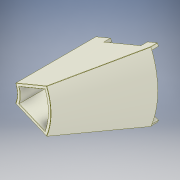
# Autodesk Inventor part: rear curved panel
Saved by Autodesk Inventor 2019 (Build 230136000, 136)
## iProperties
Created: 2019-01-04
Part Number: rear curved panel
Material: Phenolic Resin
Document SubType Name: Sheet Metal
Designer: gaincarlo
Density: 1.38 g/cm^3
Appearance: Smooth - Ivory
Sheet Metal Rule: Default_mm
Author: gaincarlo
Autodesk Inventor part; units mm, degrees
ref_plane "Work Plane1" through (0, 0, 600) normal (0, 0, 1) x (1, 0, 0)
sketch "Sketch1" plane through (0, 0, 600) normal (0, 0, 1) x (1, 0, 0)
  line L0 (-203.901986, -66.969601) -> (27.067897, -162.640459)
  arc A0 (-203.901986, -66.969601) -> (-203.901986, 66.969601) centre (-365.580904, 0) ccw
  line L1 (-203.901986, 66.969601) -> (27.067897, 162.640459)
  line L2 (-365.580904, 0) -> (376.715348, 0) construction
  arc A1 (27.067897, -162.640459) -> (27.067897, 162.640459) centre (-365.580904, 0) ccw
  point P0 (0, 0)
  dimension "d1" = 22.5
  dimension "d2" = 22.5
  dimension "d3" = 250
  dimension "d6" = 350
  constraints: 6 end point, 4 point on circle, 2 centre point, 1 coincident, 1 horizontal
  measures "d1" angle of L2 L0
  measures "d2" angle of L1 L2
  measures "d3" radial gap between concentric circles of A1 A0
  measures "d6" diameter of A0
ref_plane "Work Plane2" through (0, 0, 50) normal (0, 0, 1) x (1, 0, 0)
sketch "Sketch2" plane through (0, 0, 50) normal (0, 0, 1) x (1, 0, 0)
  circle A0 centre (-365.580904, 0) radius 175 construction
  arc A1 (258.03778, -258.311317) -> (258.03778, 258.311317) centre (-365.580904, 0) ccw
  line L0 (-203.901986, -66.969601) -> (258.03778, -258.311317)
  line L1 (-203.901986, 66.969601) -> (258.03778, 258.311317)
  arc A2 (-203.901986, -66.969601) -> (-203.901986, 66.969601) centre (-365.580904, 0) ccw
  dimension "d5" = 500
  constraints: 6 point on circle, 4 end point, 2 centre point, 1 coincident
  measures "d5" radial gap between concentric circles of A1 A0
loft "Loft1" add profiles "Sketch2", "Sketch1"
sketch "Sketch3" plane through (-365.580904, 0, 600) normal (0, 0, 1) x (1, 0, 0)
  line L0 (392.648801, -162.640459) -> (161.678918, -66.969601)
  arc A0 (161.678918, -66.969601) -> (161.678918, 66.969601) centre (0, 0) ccw
  line L1 (161.678918, 66.969601) -> (392.648801, 162.640459)
  arc A1 (392.648801, -162.640459) -> (392.648801, 162.640459) centre (0, 0) ccw
  line L2 (186.860104, -55.752145) -> (381.368364, -136.320105)
  arc A2 (381.368364, -136.320105) -> (381.368364, 136.320105) centre (0, 0) ccw
  line L3 (381.368364, 136.320105) -> (186.860104, 55.752145)
  arc A3 (186.860104, -55.752145) -> (186.860104, 55.752145) centre (0, 0) ccw
  point P0 (365.580904, 0)
  dimension "d11" = 20
  constraints: 4 end point, 4 point on circle, 2 centre point, 3 other
  measures "d11" distance between parallel lines of L0 L2
extrude "Extrusion1" cut sketch "Sketch3" against normal blind 250 contours A3 L3 A2 L2
sketch "Sketch4" plane through (-365.580904, 0, 50) normal (0, 0, -1) x (-1, 0, 0)
  line L0 (-161.678918, -66.969601) -> (-623.618684, -258.311317) construction
  arc A0 (-623.618684, 258.311317) -> (-623.618684, -258.311317) centre (0, 0) ccw construction
  line L1 (-623.618684, 258.311317) -> (-161.678918, 66.969601) construction
  arc A1 (-161.678918, 66.969601) -> (-161.678918, -66.969601) centre (0, 0) ccw construction
  line L2 (-186.860104, 55.752145) -> (-381.368364, 136.320105) construction
  arc A2 (-186.860104, 55.752145) -> (-186.860104, -55.752145) centre (0, 0) ccw construction
  line L3 (-381.368364, -136.320105) -> (-186.860104, -55.752145) construction
  line L4 (-272.544462, 112.891613) -> (-280.198131, 94.414022)
  line L5 (-173.853387, 20) -> (-193.971647, 20)
  line L6 (-272.544462, 112.891613) -> (-161.678918, 66.969601)
  line L7 (-186.860104, 55.752145) -> (-381.368364, 136.320105) construction
  line L8 (-280.198131, 94.414022) -> (-186.860104, 55.752145)
  arc A3 (-161.678918, 66.969601) -> (-161.678918, -66.969601) centre (0, 0) ccw construction
  arc A4 (-161.678918, 66.969601) -> (-173.853387, 20) centre (0, 0) ccw
  arc A5 (-186.860104, 55.752145) -> (-186.860104, -55.752145) centre (0, 0) ccw construction
  arc A6 (-186.860104, 55.752145) -> (-193.971647, 20) centre (0, 0) ccw
  line L9 (-549.708322, 227.696642) -> (-557.36199, 209.219052)
  line L10 (-557.36199, 209.219052) -> (-630.998551, 239.720314)
  line L11 (-161.678918, 66.969601) -> (-623.618684, 258.311317) construction
  arc A7 (-623.618684, 258.311317) -> (-623.618684, -258.311317) centre (0, 0) ccw construction
  arc A8 (-623.618684, 258.311317) -> (-630.998551, 239.720314) centre (0, 0) ccw
  line L12 (-623.618684, 258.311317) -> (-392.648801, 162.640459) construction
  line L13 (-623.618684, 258.311317) -> (-549.708322, 227.696642)
  point P0 (-365.580904, 0)
  dimension "d14" = 120
  dimension "d15" = 20
  dimension "d18" = 80
  dimension "d20" = 20
  constraints: 14 end point, 10 point on circle, 4 perpendicular, 3 centre point, 3 coincident, 3 point on line, 1 collinear, 1 horizontal
  measures "d14" distance from line of L4 L1.end
  measures "d15" distance from line of A0.centre L5
  measures "d18" distance from line of L9 L1.start
  measures "d20" distance of L9.start L9.end
extrude "Extrusion2" add sketch "Sketch4" along normal blind 50
mirror "Mirror1" about plane through (0, 0, 0) normal (0, 1, 0) of "Extrusion2"
ref_plane "Work Plane3" through (0, 0, 300) normal (0, 0, 1) x (1, 0, 0)
sketch "Sketch5" plane through (0, 0, 300) normal (0, 0, 1) x (1, 0, 0)
  line L0 (153.05147, -214.824563) -> (-203.901986, -66.969601) construction
  arc A0 (-203.901986, -66.969601) -> (-203.901986, 66.969601) centre (-365.580904, 0) ccw construction
  line L1 (-203.901986, 66.969601) -> (153.05147, 214.824563) construction
  arc A1 (153.05147, -214.824563) -> (153.05147, 214.824563) centre (-365.580904, 0) ccw construction
  line L2 (-166.744101, -49.889135) -> (136.032549, -175.303329)
  arc A2 (136.032549, -175.303329) -> (136.032549, 175.303329) centre (-365.580904, 0) ccw construction
  line L3 (136.032549, 175.303329) -> (-166.744101, 49.889135)
  arc A3 (-166.744101, -49.889135) -> (-166.744101, 49.889135) centre (-365.580904, 0) ccw construction
  line L4 (136.032549, -175.303329) -> (136.032549, 175.303329)
  line L5 (-166.744101, -49.889135) -> (-166.744101, 49.889135)
  point P0 (0, 0)
  dimension "d22" = 30
  constraints: 8 end point, 4 point on circle, 2 centre point, 2 vertical, 3 other
  measures "d22" distance between parallel lines of L0 L2
sketch "Sketch6" plane through (-171.609257, 20, 50) normal (0, 0, -1) x (-1, 0, 0)
  line L0 (-78.572815, -132.891613) -> (-86.226483, -114.414022) construction
  line L1 (-86.226483, -114.414022) -> (7.111544, -75.752145) construction
  arc A0 (0, -40) -> (7.111544, -75.752145) centre (193.971647, -20) ccw construction
  line L2 (0, -40) -> (20.118261, -40) construction
  arc A1 (20.118261, 0) -> (20.118261, -40) centre (193.971647, -20) ccw construction
  line L3 (20.118261, 0) -> (0, 0) construction
  arc A2 (7.111544, 35.752145) -> (0, 0) centre (193.971647, -20) ccw construction
  line L4 (7.111544, 35.752145) -> (-86.226483, 74.414022) construction
  line L5 (-86.226483, 74.414022) -> (-78.572815, 92.891613) construction
  line L6 (-78.572815, 92.891613) -> (-355.736674, 207.696642) construction
  line L7 (-355.736674, 207.696642) -> (-363.390343, 189.219052) construction
  line L8 (-363.390343, 189.219052) -> (-437.026903, 219.720314) construction
  arc A3 (-437.026903, 219.720314) -> (-437.026903, -259.720314) centre (193.971647, -20) ccw construction
  line L9 (-437.026903, -259.720314) -> (-363.390343, -229.219052) construction
  line L10 (-363.390343, -229.219052) -> (-355.736674, -247.696642) construction
  line L11 (-355.736674, -247.696642) -> (-78.572815, -132.891613) construction
  line L12 (-355.736674, 207.696642) -> (-363.390343, 189.219052) construction
  line L13 (-363.390343, 189.219052) -> (-437.026903, 219.720314) construction
  arc A4 (-429.647037, 238.311317) -> (-437.026903, 219.720314) centre (193.971647, -20) ccw construction
  line L14 (-429.647037, 238.311317) -> (-355.736674, 207.696642) construction
  line L15 (-355.736674, 207.696642) -> (-78.572815, 92.891613) construction
  line L16 (-78.572815, 92.891613) -> (32.292729, 46.969601) construction
  arc A5 (32.292729, 46.969601) -> (20.118261, 0) centre (193.971647, -20) ccw construction
  arc A6 (20.118261, 0) -> (20.118261, -40) centre (193.971647, -20) ccw construction
  arc A7 (20.118261, -40) -> (32.292729, -86.969601) centre (193.971647, -20) ccw construction
  line L17 (32.292729, -86.969601) -> (-78.572815, -132.891613) construction
  line L18 (-78.572815, -132.891613) -> (-86.226483, -114.414022) construction
  line L19 (-86.226483, -114.414022) -> (7.111544, -75.752145) construction
  arc A8 (0, -40) -> (7.111544, -75.752145) centre (193.971647, -20) ccw construction
  line L20 (0, -40) -> (20.118261, -40) construction
  arc A9 (-437.026903, 219.720314) -> (-437.026903, -259.720314) centre (193.971647, -20) ccw construction
  arc A10 (-437.026903, -259.720314) -> (-429.647037, -278.311317) centre (193.971647, -20) ccw construction
  line L21 (-355.736674, -247.696642) -> (-429.647037, -278.311317) construction
  line L22 (-363.390343, -229.219052) -> (-355.736674, -247.696642) construction
  line L23 (-437.026903, -259.720314) -> (-363.390343, -229.219052) construction
  line L24 (-86.226483, 74.414022) -> (-78.572815, 92.891613) construction
  line L25 (7.111544, 35.752145) -> (-86.226483, 74.414022) construction
  arc A11 (7.111544, 35.752145) -> (0, 0) centre (193.971647, -20) ccw construction
  line L26 (20.118261, 0) -> (0, 0) construction
  line L27 (-78.572815, -132.891613) -> (-355.736674, -247.696642) construction
  line L28 (-412.766238, -238.847295) -> (-4.865156, -69.889135)
  line L29 (-4.865156, 29.889135) -> (-412.766238, 198.847295)
  line L30 (-355.736674, 207.696642) -> (-363.390343, 189.219052) construction
  line L31 (-363.390343, 189.219052) -> (-437.026903, 219.720314) construction
  arc A12 (-429.647037, 238.311317) -> (-437.026903, 219.720314) centre (193.971647, -20) ccw construction
  line L32 (-429.647037, 238.311317) -> (-355.736674, 207.696642) construction
  line L33 (-355.736674, 207.696642) -> (-78.572815, 92.891613) construction
  line L34 (-78.572815, 92.891613) -> (32.292729, 46.969601) construction
  arc A13 (32.292729, 46.969601) -> (20.118261, 0) centre (193.971647, -20) ccw construction
  arc A14 (20.118261, 0) -> (20.118261, -40) centre (193.971647, -20) ccw construction
  arc A15 (20.118261, -40) -> (32.292729, -86.969601) centre (193.971647, -20) ccw construction
  line L35 (32.292729, -86.969601) -> (-78.572815, -132.891613) construction
  line L36 (-78.572815, -132.891613) -> (-86.226483, -114.414022) construction
  line L37 (-86.226483, -114.414022) -> (7.111544, -75.752145) construction
  arc A16 (0, -40) -> (7.111544, -75.752145) centre (193.971647, -20) ccw construction
  line L38 (0, -40) -> (20.118261, -40) construction
  arc A17 (-437.026903, 219.720314) -> (-437.026903, -259.720314) centre (193.971647, -20) ccw construction
  arc A18 (-437.026903, -259.720314) -> (-429.647037, -278.311317) centre (193.971647, -20) ccw construction
  line L39 (-355.736674, -247.696642) -> (-429.647037, -278.311317) construction
  line L40 (-363.390343, -229.219052) -> (-355.736674, -247.696642) construction
  line L41 (-437.026903, -259.720314) -> (-363.390343, -229.219052) construction
  line L42 (-86.226483, 74.414022) -> (-78.572815, 92.891613) construction
  line L43 (7.111544, 35.752145) -> (-86.226483, 74.414022) construction
  arc A19 (7.111544, 35.752145) -> (0, 0) centre (193.971647, -20) ccw construction
  line L44 (20.118261, 0) -> (0, 0) construction
  line L45 (-78.572815, -132.891613) -> (-355.736674, -247.696642) construction
  line L46 (-355.736674, 207.696642) -> (-363.390343, 189.219052) construction
  line L47 (-363.390343, 189.219052) -> (-437.026903, 219.720314) construction
  arc A20 (-429.647037, 238.311317) -> (-437.026903, 219.720314) centre (193.971647, -20) ccw construction
  line L48 (-429.647037, 238.311317) -> (-355.736674, 207.696642) construction
  line L49 (-355.736674, 207.696642) -> (-78.572815, 92.891613) construction
  line L50 (-78.572815, 92.891613) -> (32.292729, 46.969601) construction
  arc A21 (32.292729, 46.969601) -> (20.118261, 0) centre (193.971647, -20) ccw construction
  arc A22 (20.118261, 0) -> (20.118261, -40) centre (193.971647, -20) ccw construction
  arc A23 (20.118261, -40) -> (32.292729, -86.969601) centre (193.971647, -20) ccw construction
  line L51 (32.292729, -86.969601) -> (-78.572815, -132.891613) construction
  line L52 (-78.572815, -132.891613) -> (-86.226483, -114.414022) construction
  line L53 (-86.226483, -114.414022) -> (7.111544, -75.752145) construction
  arc A24 (0, -40) -> (7.111544, -75.752145) centre (193.971647, -20) ccw construction
  line L54 (0, -40) -> (20.118261, -40) construction
  arc A25 (-437.026903, 219.720314) -> (-437.026903, -259.720314) centre (193.971647, -20) ccw construction
  arc A26 (-437.026903, -259.720314) -> (-429.647037, -278.311317) centre (193.971647, -20) ccw construction
  line L55 (-355.736674, -247.696642) -> (-429.647037, -278.311317) construction
  line L56 (-363.390343, -229.219052) -> (-355.736674, -247.696642) construction
  line L57 (-437.026903, -259.720314) -> (-363.390343, -229.219052) construction
  line L58 (-86.226483, 74.414022) -> (-78.572815, 92.891613) construction
  line L59 (7.111544, 35.752145) -> (-86.226483, 74.414022) construction
  arc A27 (7.111544, 35.752145) -> (0, 0) centre (193.971647, -20) ccw construction
  line L60 (20.118261, 0) -> (0, 0) construction
  line L61 (-78.572815, -132.891613) -> (-355.736674, -247.696642) construction
  arc A28 (-9.685177, -43.428571) -> (-4.865156, -69.889135) centre (193.971647, -20) ccw construction
  arc A29 (-9.685177, 3.428571) -> (-9.685177, -43.428571) centre (193.971647, -20) ccw construction
  arc A30 (-409.297777, -248.234533) -> (-408.982523, -249.066077) centre (193.971647, -20) ccw construction
  arc A31 (-408.982523, 209.066077) -> (-409.297777, 208.234533) centre (193.971647, -20) ccw construction
  arc A32 (-412.766238, 198.847295) -> (-412.766238, -238.847295) centre (193.971647, -20) ccw construction
  arc A33 (-4.865156, 29.889135) -> (-9.685177, 3.428571) centre (193.971647, -20) ccw construction
  line L62 (-4.865156, -69.889135) -> (-4.865156, 29.889135)
  line L63 (-412.766238, -238.847295) -> (-412.766238, 198.847295)
  point P0 (-171.609257, -20)
  dimension "d24" = 30
  dimension "d25" = 30
  dimension "d26" = 30
  dimension "d27" = 30
  constraints: 12 point on circle, 8 end point, 6 centre point, 2 parallel, 2 point on line, 1 vertical
  measures "d24" distance between parallel lines of L28 L27
  measures "d25" distance between parallel lines of L29 L6
  measures "d26" radial gap between concentric circles of A29 A1
  measures "d27" radial gap between concentric circles of A28 A7
loft "Loft2" cut profiles "Sketch5", "Sketch6"
fillet "Fillet1" radius 2 16 edges at (-203.902, -66.9696, 325) (-203.902, -66.9696, 25) (-203.902, 66.9696, 325) (-203.902, 66.9696, 25) (142.5528, -210.4759, 325) (142.5528, 210.4759, 325) (-88.417, 114.805, 600) (-190.5809, 0, 600) (-88.417, -114.805, 600) (59.4191, 0, 600) (39.4191, 0, 600) (-81.4667, 96.0361, 600) (-170.5809, 0, 600) (-81.4667, -96.0361, 600) (258.0378, 258.3113, 25) (258.0378, -258.3113, 25)
thicken "Thicken1" operation new thickness 2 both sides no extend neighbours no toward (0.8502244, -0.3254007, 0.4138029) faces at (148.215845, -196.642021, 324.689671)
thicken "Thicken2" operation new thickness 2 both sides no extend neighbours no toward (-0.9990096, 0.0444948, 0) faces at (-190.754221, -7.786591, 415.333333) (-201.295818, -60.294364, 33.333333) (-195.315477, 40.43123, 33.333333)
equation "\"d2\" = d1"
equation "\"BendRadius\" = Thickness"
equation "\"BendReliefWidth\" = Thickness"
equation "\"BendReliefDepth\" = 0.5 * Thickness"
equation "\"CornerReliefSize\" = 4 * Thickness"
equation "\"MinimumRemnant\" = 2 * Thickness"
equation "\"TransitionRadius\" = BendRadius"
equation "\"JacobiRadiusSize\" = BendRadius"
equation "\"GapSize\" = Thickness"
equation "\"Thickness\" = 2"
body "Solid1"
body "Solid2"
body "Solid3"
